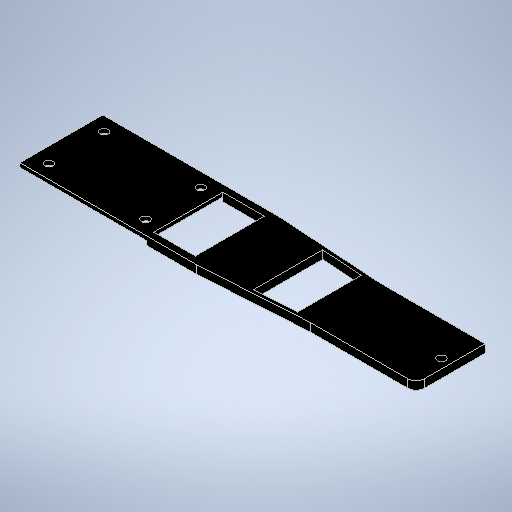
# Autodesk Inventor part: nakladka_boczna2
Saved by Autodesk Inventor 2025.2 (Build 292293000, 293)
## iProperties
Created: 2026-04-12
Part Number: nakladka_boczna2
Material: PCTG 20%
Document SubType Name: Modeling
Designer: ksawe
Density: 1.541 g/cm^3
Appearance: Anodized - Black
Author: ksawe
Autodesk Inventor part; units mm, degrees
ref_plane "YZ Plane" through (0, 0, 0) normal (1, 0, 0) x (0, 1, 0)
ref_plane "XZ Plane" through (0, 0, 0) normal (0, 1, 0) x (-1, 0, 0)
ref_plane "XY Plane" through (0, 0, 0) normal (0, 0, 1) x (1, 0, 0)
sketch "Sketch1" plane through (0, 0, 0) normal (0, 1, 0) x (-1, 0, 0)
  line L0 (-79.8192, 12.5065) -> (-40.859, 15)
  line L1 (-40.859, 15) -> (0, 15)
  line L2 (-80.022, 0) -> (80.022, 0) construction
  line L3 (-80.022, -12.4935) -> (-40.859, -15)
  line L4 (-40.859, -15) -> (0, -15)
  line L5 (0, 15) -> (0, -15) construction
  line L6 (40.859, 15) -> (0, 15)
  line L7 (79.8192, 12.5065) -> (40.859, 15)
  line L8 (80.022, -12.4935) -> (40.859, -15)
  line L9 (40.859, -15) -> (0, -15)
  line L10 (-59.1282, -12.5) -> (-74.1282, -11.54)
  line L11 (-59.1282, 12.5) -> (-74.1282, 11.54)
  line L12 (-74.1282, 11.54) -> (-74.1282, -11.54)
  line L13 (-59.1282, 12.5) -> (-59.1282, -12.5)
  line L14 (-23, 12.5) -> (-38, 12.5)
  line L15 (-38, 12.5) -> (-38, -12.5)
  line L16 (-38, -12.5) -> (-23, -12.5)
  line L17 (-23, -12.5) -> (-23, 12.5)
  line L18 (59.1282, -12.5) -> (74.1282, -11.54)
  line L19 (59.1282, 12.5) -> (74.1282, 11.54)
  line L20 (74.1282, 11.54) -> (74.1282, -11.54)
  line L21 (59.1282, 12.5) -> (59.1282, -12.5)
  line L22 (23, 12.5) -> (38, 12.5)
  line L23 (38, 12.5) -> (38, -12.5)
  line L24 (38, -12.5) -> (23, -12.5)
  line L25 (23, -12.5) -> (23, 12.5)
  circle A0 centre (-17.5, -10) radius 1.5
  circle A1 centre (17.5, -10) radius 1.5
  circle A2 centre (-17.5, 10) radius 1.5
  circle A3 centre (17.5, 10) radius 1.5
  line L26 (-79.8192, 12.5065) -> (-118.022, 12.5065)
  line L27 (-118.022, 12.5065) -> (-118.022, -12.4935)
  line L28 (-80.022, -12.4935) -> (-118.022, -12.4935)
  circle A4 centre (-114.702, 0) radius 1.5
  line L29 (79.8192, 12.5065) -> (118.022, 12.5065)
  line L30 (118.022, 12.5065) -> (118.022, -12.4935)
  line L31 (80.022, -12.4935) -> (118.022, -12.4935)
  circle A5 centre (114.702, 0) radius 1.5
  point P0 (0, 0)
  point P1 (0, 0)
  point P2 (0, 0)
  point P3 (-74.1282, 0)
  point P4 (-30.5, 12.5)
  dimension "d11" = 15
  dimension "d13" = 3
  dimension "d14" = 5
  dimension "d15" = 5.5
  dimension "d17" = 38
  dimension "d23" = 3
  dimension "d24" = 3.32
  dimension "d33" = 23
  dimension "d44" = 40.859
  dimension "d45" = 39.163
  dimension "d49" = 30
  dimension "d50" = 25
  dimension "d51" = 5.8938
  dimension "d52" = 15
  dimension "d53" = 25
  dimension "d54" = 1.328
  constraints: 64 end point, 22 symmetric about line, 6 centre point, 5 horizontal, 4 midpoint, 4 parallel, 3 coincident, 3 horizontal alignment, 2 perpendicular, 2 vertical, 1 vertical alignment, 5 other
  measures "d11" distance of L14.start L14.end
  measures "d13" diameter of A0
  measures "d14" distance from line of L4 A0.centre
  measures "d15" distance from line of L17 A0.centre
  measures "d17" distance of L3.start L27.end
  measures "d23" diameter of A4
  measures "d24" distance from line of L27 A4.centre
  measures "d33" distance from line of L17 point (0, 0)
  measures "d44" distance of L1.end L0.end
  measures "d45" horizontal distance of L3.start L3.end
  measures "d49" distance between parallel lines of L1 L4
  measures "d50" distance between parallel lines of L26 L28
  measures "d51" distance from line of L3.start L12
  measures "d52" distance from line of L12 L11.start
  measures "d53" distance from line of point (-30.5, 12.5) L16
  measures "d54" distance between parallel lines of L3 L10
extrude "Extrusion1" add sketch "Sketch1" along normal mid plane 3
fillet "Fillet1" radius 3 2 edges at (-118.022, 0, 12.5065) (118.022, 0, 12.5065)
sketch "Sketch3" plane through (-40.859, 1.5, 15) normal (0, 0, 1) x (1, 0, 0)
  line L0 (0, 0) -> (81.718, 0) projected
  line L1 (81.718, -3) -> (0, -3) projected
  line L2 (17.859, -3) -> (17.859, 0) projected
  line L3 (63.859, -3) -> (63.859, 0) projected
  line L4 (17.859, -3) -> (17.859, 0) projected
  line L5 (17.859, -1.5) -> (63.859, -1.5)
  line L6 (158.881, -3) -> (158.881, 0) projected
  line L7 (120.6782, 0) -> (155.881, 0) projected
  line L8 (155.881, 0) -> (158.881, 0) projected
  line L9 (158.881, -3) -> (155.881, -3) projected
  line L10 (155.881, -3) -> (120.6782, -3) projected
  line L11 (120.6782, -3) -> (81.718, -3) projected
  line L12 (81.718, 0) -> (120.6782, 0) projected
  line L13 (-38.9602, 0) -> (0, 0) projected
  line L14 (0, -3) -> (-38.9602, -3) projected
  line L15 (-74.163, 0) -> (-38.9602, 0) projected
  line L16 (-38.9602, -3) -> (-74.163, -3) projected
  line L17 (-77.163, 0) -> (-77.163, -3) projected
  line L18 (-74.163, -3) -> (-77.163, -3) projected
  line L19 (-77.163, 0) -> (-74.163, 0) projected
  point P0 (40.859, -1.5)
  point P1 (17.859, -1.5)
  constraints: 2 end point, 2 midpoint
extrude "Extrusion3" cut sketch "Sketch3" against normal through all contours L0 L2 L1 L14 L16 L18 L17 L19 L15 L13 | L5 L3 L1 L2
body "Solid1"
